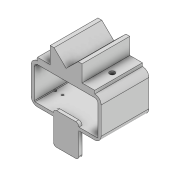
# Autodesk Inventor part: Base soporte tubos
Saved by Autodesk Inventor 2021 (Build 250183000, 183)
## iProperties
Created: 2021-04-30
Part Number: Base soporte tubos
Material: Generic
Document SubType Name: Modeling
Designer: Nelson
Density: 1 g/cm^3
Appearance: Default
Author: Nelson
Autodesk Inventor part; units mm, degrees
ref_plane "YZ Plane" through (0, 0, 0) normal (1, 0, 0) x (0, 1, 0)
ref_plane "XZ Plane" through (0, 0, 0) normal (0, 1, 0) x (-1, 0, 0)
ref_plane "XY Plane" through (0, 0, 0) normal (0, 0, 1) x (1, 0, 0)
sketch "Sketch1" plane through (0, 0, 0) normal (0, 0, 1) x (1, 0, 0)
  line L0 (-100, 0) -> (-100, 70)
  line L1 (-90, 80) -> (90, 80)
  line L2 (100, 70) -> (100, 0)
  arc A0 (-90, 80) -> (-100, 70) centre (-90, 70) ccw
  arc A1 (100, 70) -> (90, 80) centre (90, 70) ccw
  line L3 (-110, 0) -> (-110, 70)
  arc A2 (-90, 90) -> (-110, 70) centre (-90, 70) ccw
  arc A3 (110, 70) -> (90, 90) centre (90, 70) ccw
  line L4 (110, 70) -> (110, 0)
  line L5 (-90, 90) -> (-90, 100)
  line L6 (90, 90) -> (90, 100)
  line L7 (-50, 100) -> (-50, 152)
  line L8 (50, 100) -> (50, 152)
  line L9 (-38, 152) -> (0, 115)
  line L10 (0, 115) -> (38, 152)
  line L11 (-50, 152) -> (-38, 152)
  line L12 (38, 152) -> (50, 152)
  line L13 (-90, 100) -> (-50, 100)
  line L14 (50, 100) -> (90, 100)
  line L15 (-110, 0) -> (-110, -15.218)
  line L16 (-90, -35.218) -> (90, -35.218)
  line L17 (110, -15.218) -> (110, 0)
  line L18 (100, 0) -> (100, -23.218)
  line L19 (98, -25.218) -> (-98, -25.218)
  line L20 (-100, -23.218) -> (-100, 0)
  line L21 (-70, 0) -> (70, 0) construction
  arc A4 (-100, -23.218) -> (-98, -25.218) centre (-98, -23.218) ccw
  arc A5 (98, -25.218) -> (100, -23.218) centre (98, -23.218) ccw
  arc A6 (-110, -15.218) -> (-90, -35.218) centre (-90, -15.218) ccw
  arc A7 (90, -35.218) -> (110, -15.218) centre (90, -15.218) ccw
  point P0 (0, 0)
  dimension "d0" = 100
  dimension "d1" = 100
  dimension "d4" = 10
  dimension "d5" = 10
  dimension "d24" = 10
  dimension "d25" = 50
  dimension "d26" = 50
  dimension "d31" = 12
  dimension "d32" = 12
  dimension "d33" = 50
  dimension "d37" = 15
  dimension "d38" = 20
  dimension "d39" = 20
  dimension "d40" = 52
  dimension "d41" = 52
  dimension "d49" = 10
  dimension "d50" = 35.218
  dimension "d51" = 2
  dimension "d52" = 20
  dimension "d53" = 20
  dimension "d54" = 80
  dimension "d55" = 10
  dimension "d57" = 10
  constraints: 44 end point, 16 point on circle, 13 tangent, 10 perpendicular, 8 centre point, 6 vertical, 4 point on line, 2 equal radius, 1 horizontal, 1 midpoint, 1 other
  measures "d0" distance from line of point (0, 0) L0
  measures "d1" distance from line of L2 point (0, 0)
  measures "d4" radius of A0
  measures "d5" distance between parallel lines of L0 L3
  measures "d24" distance of L5.start L5.end
  measures "d25" distance from line of L7 point (0, 0)
  measures "d26" distance from line of L8 point (0, 0)
  measures "d31" distance of L7.end L9.start
  measures "d32" distance of L10.end L8.end
  measures "d33" distance from line of L7 L9.end
  measures "d37" distance from line of L14 L9.end
  measures "d38" distance between parallel lines of L1 L13
  measures "d39" distance between parallel lines of L1 L14
  measures "d40" distance between parallel lines of L13 L11
  measures "d41" distance between parallel lines of L14 L12
  measures "d49" distance between parallel lines of L19 L16
  measures "d50" distance between parallel lines of L16 L21
  measures "d51" radius of A4
  measures "d52" radius of A6
  measures "d53" radius of A7
  measures "d54" distance between parallel lines of L1 L21
  measures "d55" distance between parallel lines of L4 L2
  measures "d57" distance from line of L6.start L14
extrude "Extrusion1" add sketch "Sketch1" against normal blind 150
sketch "Sketch4" plane through (-90, 100, 0) normal (0, 1, 0) x (1, 0, 0)
  circle A0 centre (20, 75) radius 8
  circle A1 centre (160, 75) radius 8
  line L0 (0, 0) -> (0, 150) projected
  line L1 (40, 0) -> (0, 0) projected
  line L2 (180, 0) -> (180, 150) projected
  line L3 (180, 0) -> (140, 0) projected
  point P0 (90, 0)
  dimension "d42" = 16
  dimension "d43" = 20
  dimension "d44" = 20
  dimension "d45" = 75
  dimension "d46" = 75
  constraints: 2 centre point, 1 equal radius
  measures "d42" diameter of A0
  measures "d43" distance from line of A0.centre L0
  measures "d44" distance from line of L2 A1.centre
  measures "d45" distance from line of L1 A0.centre
  measures "d46" distance from line of L3 A1.centre
extrude "Extrusion4" cut sketch "Sketch4" against normal blind 50
sketch "Sketch5" plane through (-90, -35.218, 0) normal (0, -1, 0) x (1, 0, 0)
  ellipse E0 centre (185.9358, -61.829) end of major axis (189.441, -61.829) minor radius 3.5052 (189.1426, -60.4136) -> (189.1426, -63.2443) ccw projected
  ellipse E1 centre (163.0377, -61.829) end of major axis (166.5429, -61.829) minor radius 3.5052 (159.831, -63.2443) -> (159.831, -60.4136) ccw projected
  ellipse E2 centre (185.9358, -117.0359) end of major axis (189.441, -117.0359) minor radius 3.5052 (189.1426, -115.6205) -> (189.1426, -118.4512) ccw projected
  ellipse E3 centre (163.0377, -117.0359) end of major axis (166.5429, -117.0359) minor radius 3.5052 (159.831, -118.4512) -> (159.831, -115.6205) ccw projected
  circle A0 centre (185.9358, -117.0359) radius 3.5052
  circle A1 centre (163.0377, -117.0359) radius 3.5052
  circle A2 centre (185.9358, -61.829) radius 3.5052
  circle A3 centre (163.0377, -61.829) radius 3.5052
  point P0 (90, 0)
  point P1 (182.4306, -61.829)
  point P2 (182.4314, -61.7571)
  point P3 (166.5422, -61.7571)
  point P4 (166.5422, -61.9009)
  point P5 (182.4314, -117.1078)
  point P6 (182.4314, -116.964)
  point P7 (166.5422, -116.964)
  point P8 (166.5422, -117.1078)
  constraints: 4 centre point, 4 coincident, 8 other
extrude "Extrusion5" cut sketch "Sketch5" against normal blind 20
sketch "Sketch6" plane through (0, 0, 0) normal (0, 0, 1) x (1, 0, 0)
  line L0 (-40, -115.218) -> (40, -115.218)
  line L1 (40, -115.218) -> (40, -15.218)
  line L2 (40, -15.218) -> (-40, -15.218)
  line L3 (-40, -15.218) -> (-40, -115.218)
  line L4 (-40, -115.218) -> (40, -15.218) construction
  line L5 (40, -115.218) -> (-40, -15.218) construction
  line L6 (98, -25.218) -> (-98, -25.218) projected
  point P0 (0, 0)
  point P1 (0, -65.218)
  point P2 (0, -65.218)
  dimension "d60" = 40
  dimension "d61" = 80
  dimension "d62" = 50
  constraints: 12 end point, 3 midpoint, 2 parallel, 1 horizontal, 1 perpendicular, 1 vertical alignment
  measures "d60" distance from line of L6 point (0, -65.218)
  measures "d61" distance of L0.start L0.end
  measures "d62" distance from line of point (0, -65.218) L2
extrude "Extrusion6" add sketch "Sketch6" against normal blind 10
fillet "Fillet2" radius 10 4 edges at (40, -15.218, -5) (-40, -15.218, -5) (40, -115.218, -5) (-40, -115.218, -5)
mirror "Mirror1" about plane through (0, 0, 0) normal (1, 0, 0) of "Extrusion5"
equation "\"d26\" = d25"
equation "\"d33\" = d25"
equation "\"d39\" = d38"
equation "\"d41\" = d40"
equation "\"d49\" = d5"
equation "\"d55\" = d5"
equation "\"d57\" = d24"
equation "\"d44\" = d43"
equation "\"d46\" = d45"
equation "\"d36\" = d34"
equation "\"d34\" = 75"
body "Solid1"
